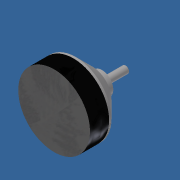
# Autodesk Inventor part: Wirnik
Saved by Autodesk Inventor 2014 SP1 (Build 180222100, 222)
## iProperties
Created: 2014-09-01
Part Number: Wirnik
Material: Stal nierdzewna
Document SubType Name: Modeling
Designer: Marcin
Density: 8.08 g/cm^3
Appearance: Częściowo polerowany
Author: Marcin
Autodesk Inventor part; units mm, degrees
ref_plane "YZ Plane" through (0, 0, 0) normal (1, 0, 0) x (0, 1, 0)
ref_plane "XZ Plane" through (0, 0, 0) normal (0, 1, 0) x (-1, 0, 0)
ref_plane "XY Plane" through (0, 0, 0) normal (0, 0, 1) x (1, 0, 0)
sketch "Szkic1" plane through (0, 0, 0) normal (0, 1, 0) x (-1, 0, 0)
  circle A0 centre (0, 0) radius 15
  dimension "d0" = 30
  constraints: 1 centre point, 1 coincident
  measures "d0" diameter of A0
extrude "Wyciągnięcie proste1" add sketch "Szkic1" along normal blind 8
sketch "Szkic2" plane through (0, 8, 0) normal (0, 1, 0) x (1, 0, 0)
  circle A0 centre (0, 0) radius 15 projected
extrude "Wyciągnięcie proste2" add sketch "Szkic2" along normal blind 8 separate body
chamfer "Faza1" distance 7 angle 45 1 edges at (-15, 16, 0)
sketch "Szkic3" plane through (0, 16, 0) normal (0, 1, 0) x (1, 0, 0)
  circle A0 centre (0, 0) radius 8 projected
  circle A1 centre (0, 0) radius 4.75
  dimension "d8" = 9.5
  constraints: 1 centre point, 1 coincident
  measures "d8" diameter of A1
extrude "Wyciągnięcie proste3" add sketch "Szkic3" along normal blind 4 contours A1 bodies 2
fillet "Zaokrąglenie1" radius 0.25 1 edges at (-4.75, 16, 0)
fillet "Zaokrąglenie2" radius 0.25 2 edges at (-15, 9, 0) (-8, 16, 0)
sketch "Szkic4" plane through (0, 20, 0) normal (0, 1, 0) x (1, 0, 0)
  circle A0 centre (0, 0) radius 4.75 projected
  circle A1 centre (0, 0) radius 1.5
  dimension "d13" = 3
  constraints: 1 centre point, 1 coincident
  measures "d13" diameter of A1
extrude "Wyciągnięcie proste4" add sketch "Szkic4" along normal blind 10 contours A1 bodies 2
fillet "Zaokrąglenie3" radius 0.25 2 edges at (-1.5, 20, 0) (-1.5, 30, 0)
